Autodesk Inventor part; units mm, degrees
(part 2 of 2)
sketch "Sketch6" plane through (4200, 27800, -3800) normal (0, 0, 1) x (1, 0, 0)
  line L0 (0, -26000) -> (1000, -26000)
  line L1 (1000, -26000) -> (1000, -26050)
  line L2 (1000, -26050) -> (0, -26050)
  line L3 (0, -26050) -> (0, -26000)
  line L4 (1000, -25800) -> (1300, -25800)
  line L5 (1300, -25800) -> (1300, -25850)
  line L6 (1300, -25850) -> (1000, -25850)
  line L7 (1000, -25850) -> (1000, -25800)
  line L8 (1300, -25600) -> (1600, -25600)
  line L9 (1600, -25600) -> (1600, -25650)
  line L10 (1600, -25650) -> (1300, -25650)
  line L11 (1300, -25650) -> (1300, -25600)
  line L12 (1600, -25400) -> (1900, -25400)
  line L13 (1900, -25400) -> (1900, -25450)
  line L14 (1900, -25450) -> (1600, -25450)
  line L15 (1600, -25450) -> (1600, -25400)
  line L16 (1900, -25200) -> (2200, -25200)
  line L17 (2200, -25200) -> (2200, -25250)
  line L18 (2200, -25250) -> (1900, -25250)
  line L19 (1900, -25250) -> (1900, -25200)
  line L20 (2200, -25000) -> (2500, -25000)
  line L21 (2500, -25000) -> (2500, -25050)
  line L22 (2500, -25050) -> (2200, -25050)
  line L23 (2200, -25050) -> (2200, -25000)
  line L24 (2500, -24800) -> (2800, -24800)
  line L25 (2800, -24800) -> (2800, -24850)
  line L26 (2800, -24850) -> (2500, -24850)
  line L27 (2500, -24850) -> (2500, -24800)
  line L28 (2800, -24600) -> (3100, -24600)
  line L29 (3100, -24600) -> (3100, -24650)
  line L30 (3100, -24650) -> (2800, -24650)
  line L31 (2800, -24650) -> (2800, -24600)
  line L32 (3100, -24400) -> (3400, -24400)
  line L33 (3400, -24400) -> (3400, -24450)
  line L34 (3400, -24450) -> (3100, -24450)
  line L35 (3100, -24450) -> (3100, -24400)
  line L36 (0, -22400) -> (1000, -22400)
  line L37 (1000, -22400) -> (1000, -22450)
  line L38 (1000, -22450) -> (0, -22450)
  line L39 (0, -22450) -> (0, -22400)
  line L40 (1000, -22200) -> (1300, -22200)
  line L41 (1300, -22200) -> (1300, -22250)
  line L42 (1300, -22250) -> (1000, -22250)
  line L43 (1000, -22250) -> (1000, -22200)
  line L44 (1300, -22000) -> (1600, -22000)
  line L45 (1600, -22000) -> (1600, -22050)
  line L46 (1600, -22050) -> (1300, -22050)
  line L47 (1300, -22050) -> (1300, -22000)
  line L48 (1600, -21800) -> (1900, -21800)
  line L49 (1900, -21800) -> (1900, -21850)
  line L50 (1900, -21850) -> (1600, -21850)
  line L51 (1600, -21850) -> (1600, -21800)
  line L52 (1900, -21600) -> (2200, -21600)
  line L53 (2200, -21600) -> (2200, -21650)
  line L54 (2200, -21650) -> (1900, -21650)
  line L55 (1900, -21650) -> (1900, -21600)
  line L56 (2200, -21400) -> (2500, -21400)
  line L57 (2500, -21400) -> (2500, -21450)
  line L58 (2500, -21450) -> (2200, -21450)
  line L59 (2200, -21450) -> (2200, -21400)
  line L60 (2500, -21200) -> (2800, -21200)
  line L61 (2800, -21200) -> (2800, -21250)
  line L62 (2800, -21250) -> (2500, -21250)
  line L63 (2500, -21250) -> (2500, -21200)
  line L64 (2800, -21000) -> (3100, -21000)
  line L65 (3100, -21000) -> (3100, -21050)
  line L66 (3100, -21050) -> (2800, -21050)
  line L67 (2800, -21050) -> (2800, -21000)
  line L68 (3100, -20800) -> (3400, -20800)
  line L69 (3400, -20800) -> (3400, -20850)
  line L70 (3400, -20850) -> (3100, -20850)
  line L71 (3100, -20850) -> (3100, -20800)
  line L72 (0, -19400) -> (1100, -19400)
  line L73 (1100, -19400) -> (1100, -19450)
  line L74 (1100, -19450) -> (0, -19450)
  line L75 (0, -19450) -> (0, -19400)
  line L76 (1100, -19250) -> (1100, -19200)
  line L77 (1400, -19250) -> (1100, -19250)
  line L78 (1100, -19200) -> (1400, -19200)
  line L79 (1400, -19200) -> (1400, -19250)
  line L80 (1400, -19050) -> (1400, -19000)
  line L81 (1700, -19050) -> (1400, -19050)
  line L82 (1400, -19000) -> (1700, -19000)
  line L83 (1700, -19000) -> (1700, -19050)
  line L84 (1700, -18794.0956) -> (1700, -18744.0956)
  line L85 (2000, -18794.0956) -> (1700, -18794.0956)
  line L86 (1700, -18744.0956) -> (2000, -18744.0956)
  line L87 (2000, -18744.0956) -> (2000, -18794.0956)
  line L88 (2000, -18594.0956) -> (2000, -18544.0956)
  line L89 (2300, -18594.0956) -> (2000, -18594.0956)
  line L90 (2000, -18544.0956) -> (2300, -18544.0956)
  line L91 (2300, -18544.0956) -> (2300, -18594.0956)
  line L92 (2300, -18394.0956) -> (2300, -18344.0956)
  line L93 (2600, -18394.0956) -> (2300, -18394.0956)
  line L94 (2300, -18344.0956) -> (2600, -18344.0956)
  line L95 (2600, -18344.0956) -> (2600, -18394.0956)
  line L96 (0, -16800) -> (1100, -16800)
  line L97 (1100, -16800) -> (1100, -16850)
  line L98 (1100, -16850) -> (0, -16850)
  line L99 (0, -16850) -> (0, -16800)
  line L100 (1100, -16650) -> (1100, -16600)
  line L101 (1400, -16650) -> (1100, -16650)
  line L102 (1100, -16600) -> (1400, -16600)
  line L103 (1400, -16600) -> (1400, -16650)
  line L104 (1400, -16450) -> (1400, -16400)
  line L105 (1700, -16450) -> (1400, -16450)
  line L106 (1400, -16400) -> (1700, -16400)
  line L107 (1700, -16400) -> (1700, -16450)
  line L108 (1700, -16194.0956) -> (1700, -16144.0956)
  line L109 (2000, -16194.0956) -> (1700, -16194.0956)
  line L110 (1700, -16144.0956) -> (2000, -16144.0956)
  line L111 (2000, -16144.0956) -> (2000, -16194.0956)
  line L112 (2000, -15994.0956) -> (2000, -15944.0956)
  line L113 (2300, -15994.0956) -> (2000, -15994.0956)
  line L114 (2000, -15944.0956) -> (2300, -15944.0956)
  line L115 (2300, -15944.0956) -> (2300, -15994.0956)
  line L116 (2300, -15794.0956) -> (2300, -15744.0956)
  line L117 (2600, -15794.0956) -> (2300, -15794.0956)
  line L118 (2300, -15744.0956) -> (2600, -15744.0956)
  line L119 (2600, -15744.0956) -> (2600, -15794.0956)
  line L120 (0, -14200) -> (1100, -14200)
  line L121 (1100, -14200) -> (1100, -14250)
  line L122 (1100, -14250) -> (0, -14250)
  line L123 (0, -14250) -> (0, -14200)
  line L124 (1100, -14050) -> (1100, -14000)
  line L125 (1400, -14050) -> (1100, -14050)
  line L126 (1100, -14000) -> (1400, -14000)
  line L127 (1400, -14000) -> (1400, -14050)
  line L128 (1400, -13850) -> (1400, -13800)
  line L129 (1700, -13850) -> (1400, -13850)
  line L130 (1400, -13800) -> (1700, -13800)
  line L131 (1700, -13800) -> (1700, -13850)
  line L132 (1700, -13594.0956) -> (1700, -13544.0956)
  line L133 (2000, -13594.0956) -> (1700, -13594.0956)
  line L134 (1700, -13544.0956) -> (2000, -13544.0956)
  line L135 (2000, -13544.0956) -> (2000, -13594.0956)
  line L136 (2000, -13394.0956) -> (2000, -13344.0956)
  line L137 (2300, -13394.0956) -> (2000, -13394.0956)
  line L138 (2000, -13344.0956) -> (2300, -13344.0956)
  line L139 (2300, -13344.0956) -> (2300, -13394.0956)
  line L140 (2300, -13194.0956) -> (2300, -13144.0956)
  line L141 (2600, -13194.0956) -> (2300, -13194.0956)
  line L142 (2300, -13144.0956) -> (2600, -13144.0956)
  line L143 (2600, -13144.0956) -> (2600, -13194.0956)
  line L144 (0, -11600) -> (1100, -11600)
  line L145 (1100, -11600) -> (1100, -11650)
  line L146 (1100, -11650) -> (0, -11650)
  line L147 (0, -11650) -> (0, -11600)
  line L148 (1100, -11450) -> (1100, -11400)
  line L149 (1400, -11450) -> (1100, -11450)
  line L150 (1100, -11400) -> (1400, -11400)
  line L151 (1400, -11400) -> (1400, -11450)
  line L152 (1400, -11250) -> (1400, -11200)
  line L153 (1700, -11250) -> (1400, -11250)
  line L154 (1400, -11200) -> (1700, -11200)
  line L155 (1700, -11200) -> (1700, -11250)
  line L156 (1700, -10994.0956) -> (1700, -10944.0956)
  line L157 (2000, -10994.0956) -> (1700, -10994.0956)
  line L158 (1700, -10944.0956) -> (2000, -10944.0956)
  line L159 (2000, -10944.0956) -> (2000, -10994.0956)
  line L160 (2000, -10794.0956) -> (2000, -10744.0956)
  line L161 (2300, -10794.0956) -> (2000, -10794.0956)
  line L162 (2000, -10744.0956) -> (2300, -10744.0956)
  line L163 (2300, -10744.0956) -> (2300, -10794.0956)
  line L164 (2300, -10594.0956) -> (2300, -10544.0956)
  line L165 (2600, -10594.0956) -> (2300, -10594.0956)
  line L166 (2300, -10544.0956) -> (2600, -10544.0956)
  line L167 (2600, -10544.0956) -> (2600, -10594.0956)
  line L168 (1700, -8650) -> (1400, -8650)
  line L169 (1700, -8600) -> (1700, -8650)
  line L170 (1400, -8650) -> (1400, -8600)
  line L171 (1400, -8600) -> (1700, -8600)
  line L172 (2000, -8394.0956) -> (1700, -8394.0956)
  line L173 (2000, -8344.0956) -> (2000, -8394.0956)
  line L174 (1700, -8394.0956) -> (1700, -8344.0956)
  line L175 (1700, -8344.0956) -> (2000, -8344.0956)
  line L176 (2000, -8194.0956) -> (2000, -8144.0956)
  line L177 (2300, -8194.0956) -> (2000, -8194.0956)
  line L178 (2000, -8144.0956) -> (2300, -8144.0956)
  line L179 (2300, -8144.0956) -> (2300, -8194.0956)
  line L180 (2300, -7994.0956) -> (2300, -7944.0956)
  line L181 (2300, -7944.0956) -> (2600, -7944.0956)
  line L182 (2600, -7944.0956) -> (2600, -7994.0956)
  line L183 (2600, -7994.0956) -> (2300, -7994.0956)
  line L184 (1400, -8800) -> (1400, -8850)
  line L185 (1100, -8800) -> (1400, -8800)
  line L186 (1100, -8850) -> (1100, -8800)
  line L187 (1400, -8850) -> (1100, -8850)
  line L188 (1100, -9000) -> (1100, -9050)
  line L189 (0, -9000) -> (1100, -9000)
  line L190 (1100, -9050) -> (0, -9050)
  line L191 (0, -9050) -> (0, -9000)
  line L192 (1700, -6050) -> (1400, -6050)
  line L193 (1700, -6000) -> (1700, -6050)
  line L194 (1400, -6050) -> (1400, -6000)
  line L195 (1400, -6000) -> (1700, -6000)
  line L196 (2000, -5794.0956) -> (1700, -5794.0956)
  line L197 (2000, -5744.0956) -> (2000, -5794.0956)
  line L198 (1700, -5794.0956) -> (1700, -5744.0956)
  line L199 (1700, -5744.0956) -> (2000, -5744.0956)
  line L200 (2000, -5594.0956) -> (2000, -5544.0956)
  line L201 (2300, -5594.0956) -> (2000, -5594.0956)
  line L202 (2000, -5544.0956) -> (2300, -5544.0956)
  line L203 (2300, -5544.0956) -> (2300, -5594.0956)
  line L204 (2300, -5394.0956) -> (2300, -5344.0956)
  line L205 (2300, -5344.0956) -> (2600, -5344.0956)
  line L206 (2600, -5344.0956) -> (2600, -5394.0956)
  line L207 (2600, -5394.0956) -> (2300, -5394.0956)
  line L208 (1400, -6200) -> (1400, -6250)
  line L209 (1100, -6200) -> (1400, -6200)
  line L210 (1100, -6250) -> (1100, -6200)
  line L211 (1400, -6250) -> (1100, -6250)
  line L212 (1100, -6400) -> (1100, -6450)
  line L213 (0, -6400) -> (1100, -6400)
  line L214 (1100, -6450) -> (0, -6450)
  line L215 (0, -6450) -> (0, -6400)
  line L216 (1700, -3450) -> (1400, -3450)
  line L217 (1700, -3400) -> (1700, -3450)
  line L218 (1400, -3450) -> (1400, -3400)
  line L219 (1400, -3400) -> (1700, -3400)
  line L220 (2000, -3194.0956) -> (1700, -3194.0956)
  line L221 (2000, -3144.0956) -> (2000, -3194.0956)
  line L222 (1700, -3194.0956) -> (1700, -3144.0956)
  line L223 (1700, -3144.0956) -> (2000, -3144.0956)
  line L224 (2000, -2994.0956) -> (2000, -2944.0956)
  line L225 (2300, -2994.0956) -> (2000, -2994.0956)
  line L226 (2000, -2944.0956) -> (2300, -2944.0956)
  line L227 (2300, -2944.0956) -> (2300, -2994.0956)
  line L228 (2300, -2794.0956) -> (2300, -2744.0956)
  line L229 (2300, -2744.0956) -> (2600, -2744.0956)
  line L230 (2600, -2744.0956) -> (2600, -2794.0956)
  line L231 (2600, -2794.0956) -> (2300, -2794.0956)
  line L232 (1400, -3600) -> (1400, -3650)
  line L233 (1100, -3600) -> (1400, -3600)
  line L234 (1100, -3650) -> (1100, -3600)
  line L235 (1400, -3650) -> (1100, -3650)
  line L236 (1100, -3800) -> (1100, -3850)
  line L237 (0, -3800) -> (1100, -3800)
  line L238 (1100, -3850) -> (0, -3850)
  line L239 (0, -3850) -> (0, -3800)
  point P0 (-4200, -27800)
  dimension "d407" = 4200
  dimension "d408" = 1800
  dimension "d409" = 50
  dimension "d410" = 1000
  dimension "d411" = 50
  dimension "d412" = 0
  dimension "d413" = 200
  dimension "d414" = 50
  dimension "d415" = 50
  dimension "d416" = 50
  dimension "d417" = 50
  dimension "d418" = 50
  dimension "d419" = 50
  dimension "d420" = 50
  dimension "d421" = 200
  dimension "d422" = 0
  dimension "d423" = 300
  dimension "d424" = 300
  dimension "d425" = 0
  dimension "d426" = 200
  dimension "d427" = 300
  dimension "d428" = 300
  dimension "d429" = 200
  dimension "d430" = 300
  dimension "d431" = 0
  dimension "d432" = 200
  dimension "d433" = 300
  dimension "d434" = 200
  dimension "d435" = 0
  dimension "d436" = 300
  dimension "d437" = 200
  dimension "d438" = 0
  dimension "d439" = 300
  dimension "d440" = 0
  dimension "d441" = 200
  dimension "d442" = 300
  dimension "d443" = 50
  dimension "d444" = 1000
  dimension "d445" = 50
  dimension "d446" = 0
  dimension "d447" = 200
  dimension "d448" = 50
  dimension "d449" = 50
  dimension "d450" = 50
  dimension "d451" = 50
  dimension "d452" = 50
  dimension "d453" = 50
  dimension "d454" = 50
  dimension "d455" = 200
  dimension "d456" = 0
  dimension "d457" = 300
  dimension "d458" = 300
  dimension "d459" = 0
  dimension "d460" = 200
  dimension "d461" = 300
  dimension "d462" = 300
  dimension "d463" = 200
  dimension "d464" = 300
  dimension "d465" = 0
  dimension "d466" = 200
  dimension "d467" = 300
  dimension "d468" = 200
  dimension "d469" = 0
  dimension "d470" = 300
  constraints: 480 end point, 120 parallel, 60 horizontal, 60 perpendicular
  measures "d407" distance from line of point (-4200, -27800) L3
  measures "d408" distance from line of point (-4200, -27800) L0
  measures "d409" distance between parallel lines of L2 L0
  measures "d410" distance between parallel lines of L3 L1
  measures "d411" distance between parallel lines of L6 L4
  measures "d412" distance between parallel lines of L1 L7
  measures "d413" distance between parallel lines of L0 L4
  measures "d414" distance between parallel lines of L10 L8
  measures "d415" distance between parallel lines of L14 L12
  measures "d416" distance between parallel lines of L18 L16
  measures "d417" distance between parallel lines of L22 L20
  measures "d418" distance between parallel lines of L26 L24
  measures "d419" distance between parallel lines of L30 L28
  measures "d420" distance between parallel lines of L34 L32
  measures "d421" distance between parallel lines of L4 L8
  measures "d422" distance between parallel lines of L5 L11
  measures "d423" distance between parallel lines of L5 L9
  measures "d424" distance between parallel lines of L7 L11
  measures "d425" distance between parallel lines of L9 L15
  measures "d426" distance between parallel lines of L8 L12
  measures "d427" distance between parallel lines of L15 L19
  measures "d428" distance between parallel lines of L9 L13
  measures "d429" distance between parallel lines of L12 L16
  measures "d430" distance between parallel lines of L13 L17
  measures "d431" distance between parallel lines of L17 L23
  measures "d432" distance between parallel lines of L16 L20
  measures "d433" distance between parallel lines of L17 L21
  measures "d434" distance between parallel lines of L20 L24
  measures "d435" distance between parallel lines of L21 L27
  measures "d436" distance between parallel lines of L21 L25
  measures "d437" distance between parallel lines of L24 L28
  measures "d438" distance between parallel lines of L25 L31
  measures "d439" distance between parallel lines of L25 L29
  measures "d440" distance between parallel lines of L35 L29
  measures "d441" distance between parallel lines of L28 L32
  measures "d442" distance between parallel lines of L29 L33
  measures "d443" distance between parallel lines of L38 L36
  measures "d444" distance between parallel lines of L39 L37
  measures "d445" distance between parallel lines of L42 L40
  measures "d446" distance between parallel lines of L37 L43
  measures "d447" distance between parallel lines of L36 L40
  measures "d448" distance between parallel lines of L46 L44
  measures "d449" distance between parallel lines of L50 L48
  measures "d450" distance between parallel lines of L54 L52
  measures "d451" distance between parallel lines of L58 L56
  measures "d452" distance between parallel lines of L62 L60
  measures "d453" distance between parallel lines of L66 L64
  measures "d454" distance between parallel lines of L70 L68
  measures "d455" distance between parallel lines of L40 L44
  measures "d456" distance between parallel lines of L41 L47
  measures "d457" distance between parallel lines of L41 L45
  measures "d458" distance between parallel lines of L43 L47
  measures "d459" distance between parallel lines of L45 L51
  measures "d460" distance between parallel lines of L44 L48
  measures "d461" distance between parallel lines of L51 L55
  measures "d462" distance between parallel lines of L45 L49
  measures "d463" distance between parallel lines of L48 L52
  measures "d464" distance between parallel lines of L49 L53
  measures "d465" distance between parallel lines of L53 L59
  measures "d466" distance between parallel lines of L52 L56
  measures "d467" distance between parallel lines of L53 L57
  measures "d468" distance between parallel lines of L56 L60
  measures "d469" distance between parallel lines of L57 L63
  measures "d470" distance between parallel lines of L57 L61
extrude "Extrusion21" add sketch "Sketch6" along normal blind 1200 and the other way blind 100 contours L0 L1 L2 L3 | L36 L37 L38 L39 | L72 L73 L74 L75 | L96 L97 L98 L99 | L120 L121 L122 L123 | L144 L145 L146 L147 | L188 L190 L191 L189 | L212 L214 L215 L213 | L236 L238 L239 L237
extrude "Extrusion22" add sketch "Sketch6" along normal blind 1200 contours L4 L5 L6 L7 | L8 L9 L10 L11 | L12 L13 L14 L15 | L16 L17 L18 L19 | L20 L21 L22 L23 | L24 L25 L26 L27 | L28 L29 L30 L31 | L32 L33 L34 L35 | L40 L41 L42 L43 | L44 L45 L46 L47 | L48 L49 L50 L51 | L52 L53 L54 L55 | L56 L57 L58 L59 | L60 L61 L62 L63 | L64 L65 L66 L67 | L68 L69 L70 L71 | L76 L78 L79 L77 | L80 L82 L83 L81 | L84 L86 L87 L85 | L88 L90 L91 L89 | L92 L94 L95 L93 | L100 L102 L103 L101 | L104 L106 L107 L105 | L108 L110 L111 L109 | L112 L114 L115 L113 | L116 L118 L119 L117 | L124 L126 L127 L125 | L128 L130 L131 L129 | L132 L134 L135 L133 | L136 L138 L139 L137 | L140 L142 L143 L141 | L148 L150 L151 L149 | L152 L154 L155 L153 | L156 L158 L159 L157 | L160 L162 L163 L161 | L164 L166 L167 L165 | L168 L170 L171 L169 | L172 L174 L175 L173 | L176 L178 L179 L177 | L180 L181 L182 L183 | L184 L187 L186 L185 | L192 L194 L195 L193 | L196 L198 L199 L197 | L200 L202 L203 L201 | L204 L205 L206 L207 | L208 L211 L210 L209 | L216 L218 L219 L217 | L220 L222 L223 L221 | L224 L226 L227 L225 | L228 L229 L230 L231 | L232 L235 L234 L233
sketch "Sketch7" plane through (11900, 0, -2400) normal (1, 0, 0) x (0, 0, -1)
  line L0 (0, 0) -> (6500, 0) projected
  line L1 (200, 2100) -> (1100, 2100)
  line L2 (1100, 2100) -> (1100, 0)
  line L3 (1100, 0) -> (200, 0)
  line L4 (200, 0) -> (200, 2100)
  line L5 (200, 5700) -> (1100, 5700)
  line L6 (1100, 5700) -> (1100, 3600)
  line L7 (1100, 3600) -> (200, 3600)
  line L8 (200, 3600) -> (200, 5700)
  line L9 (200, 9300) -> (1100, 9300)
  line L10 (1100, 9300) -> (1100, 7200)
  line L11 (1100, 7200) -> (200, 7200)
  line L12 (200, 7200) -> (200, 9300)
  line L13 (200, 11900) -> (1100, 11900)
  line L14 (1100, 11900) -> (1100, 9800)
  line L15 (1100, 9800) -> (200, 9800)
  line L16 (200, 9800) -> (200, 11900)
  line L17 (200, 14500) -> (1100, 14500)
  line L18 (1100, 14500) -> (1100, 12400)
  line L19 (1100, 12400) -> (200, 12400)
  line L20 (200, 12400) -> (200, 14500)
  line L21 (200, 17100) -> (1100, 17100)
  line L22 (1100, 17100) -> (1100, 15000)
  line L23 (1100, 15000) -> (200, 15000)
  line L24 (200, 15000) -> (200, 17100)
  line L25 (200, 19700) -> (1100, 19700)
  line L26 (1100, 19700) -> (1100, 17600)
  line L27 (1100, 17600) -> (200, 17600)
  line L28 (200, 17600) -> (200, 19700)
  line L29 (200, 22300) -> (1100, 22300)
  line L30 (1100, 22300) -> (1100, 20200)
  line L31 (1100, 20200) -> (200, 20200)
  line L32 (200, 20200) -> (200, 22300)
  line L33 (200, 24900) -> (1100, 24900)
  line L34 (1100, 24900) -> (1100, 22800)
  line L35 (1100, 22800) -> (200, 22800)
  line L36 (200, 22800) -> (200, 24900)
  line L37 (200, 27500) -> (1100, 27500)
  line L38 (1100, 27500) -> (1100, 25400)
  line L39 (1100, 25400) -> (200, 25400)
  line L40 (200, 25400) -> (200, 27500)
  point P0 (-2400, 0)
  dimension "d653" = 2600
  dimension "d654" = 0
  dimension "d655" = 2100
  dimension "d656" = 900
  dimension "d657" = 900
  dimension "d658" = 1500
  dimension "d659" = 900
  dimension "d660" = 2100
  dimension "d661" = 900
  dimension "d662" = 2100
  dimension "d663" = 900
  dimension "d664" = 2100
  dimension "d665" = 900
  dimension "d666" = 2100
  dimension "d667" = 900
  dimension "d668" = 2100
  dimension "d669" = 900
  dimension "d670" = 2100
  dimension "d671" = 900
  dimension "d672" = 2100
  dimension "d673" = 900
  dimension "d674" = 2100
  dimension "d675" = 900
  dimension "d676" = 2100
  dimension "d677" = 7200
  dimension "d678" = 2600
  dimension "d679" = 2600
  dimension "d680" = 900
  dimension "d681" = 2600
  dimension "d682" = 900
  dimension "d683" = 2600
  dimension "d684" = 900
  dimension "d685" = 2600
  dimension "d686" = 900
  dimension "d687" = 2600
  dimension "d688" = 900
  dimension "d689" = 2600
  dimension "d690" = 900
  dimension "d691" = 2600
  dimension "d692" = 900
  dimension "d693" = 900
  constraints: 80 end point, 20 parallel, 10 horizontal, 10 perpendicular
  measures "d653" distance from line of L4 point (-2400, 0)
  measures "d654" distance from line of point (-2400, 0) L3
  measures "d655" distance between parallel lines of L0 L1
  measures "d656" distance between parallel lines of L2 L4
  measures "d657" distance between parallel lines of L6 L8
  measures "d658" distance between parallel lines of L1 L7
  measures "d659" distance between parallel lines of L4 L6
  measures "d660" distance between parallel lines of L5 L7
  measures "d661" distance between parallel lines of L10 L12
  measures "d662" distance between parallel lines of L9 L11
  measures "d663" distance between parallel lines of L14 L16
  measures "d664" distance between parallel lines of L13 L15
  measures "d665" distance between parallel lines of L18 L20
  measures "d666" distance between parallel lines of L17 L19
  measures "d667" distance between parallel lines of L22 L24
  measures "d668" distance between parallel lines of L21 L23
  measures "d669" distance between parallel lines of L26 L28
  measures "d670" distance between parallel lines of L25 L27
  measures "d671" distance between parallel lines of L30 L32
  measures "d672" distance between parallel lines of L29 L31
  measures "d673" distance between parallel lines of L34 L36
  measures "d674" distance between parallel lines of L33 L35
  measures "d675" distance between parallel lines of L38 L40
  measures "d676" distance between parallel lines of L37 L39
  measures "d677" distance from line of point (-2400, 0) L11
  measures "d678" distance from line of point (-2400, 0) L12
  measures "d679" distance between parallel lines of L9 L13
  measures "d680" distance between parallel lines of L10 L16
  measures "d681" distance between parallel lines of L17 L13
  measures "d682" distance between parallel lines of L14 L20
  measures "d683" distance between parallel lines of L21 L17
  measures "d684" distance between parallel lines of L18 L24
  measures "d685" distance between parallel lines of L21 L25
  measures "d686" distance between parallel lines of L22 L28
  measures "d687" distance between parallel lines of L25 L29
  measures "d688" distance between parallel lines of L26 L32
  measures "d689" distance between parallel lines of L29 L33
  measures "d690" distance between parallel lines of L30 L36
  measures "d691" distance between parallel lines of L33 L37
  measures "d692" distance between parallel lines of L34 L40
  measures "d693" distance between parallel lines of L6 L12
extrude "Extrusion23" cut sketch "Sketch7" against normal blind 200 contours L4 L1 L2 L0
extrude "Extrusion24" cut sketch "Sketch7" against normal blind 200 contours L5 L6 L7 L8
extrude "Extrusion25" cut sketch "Sketch7" against normal blind 200 contours L9 L10 L11 L12 | L13 L14 L15 L16 | L17 L18 L19 L20 | L21 L22 L23 L24 | L25 L26 L27 L28 | L29 L30 L31 L32 | L33 L34 L35 L36 | L37 L38 L39 L40
sketch "Sketch9" plane through (4200, 27800, -3900) normal (0, 0, 1) x (1, 0, 0)
  line L0 (0, -24200) -> (3400, -24200)
  line L1 (3400, -24200) -> (3400, -24400)
  line L2 (3400, -24400) -> (0, -24400)
  line L3 (0, -24400) -> (0, -24200)
  point P0 (-4200, -27800)
  dimension "d742" = 4200
  dimension "d743" = 3400
  dimension "d744" = 200
  dimension "d745" = 3400
  constraints: 8 end point, 2 parallel, 1 horizontal, 1 perpendicular
  measures "d742" distance from line of point (-4200, -27800) L3
  measures "d743" distance from line of point (-4200, -27800) L2
  measures "d744" distance between parallel lines of L2 L0
  measures "d745" distance between parallel lines of L3 L1
extrude "Extrusion27" cut sketch "Sketch9" along normal blind 1300 and the other way blind 1200
sketch "Sketch10" plane through (4200, 27800, -3900) normal (0, 0, 1) x (1, 0, 0)
  line L0 (0, -20600) -> (3400, -20600)
  line L1 (3400, -20600) -> (3400, -20800)
  line L2 (3400, -20800) -> (0, -20800)
  line L3 (0, -20800) -> (0, -20600)
  line L4 (0, -18000) -> (2600, -18000)
  line L5 (2600, -18000) -> (2600, -18200)
  line L6 (2600, -18200) -> (0, -18200)
  line L7 (0, -18200) -> (0, -18000)
  line L8 (0, -15400) -> (2600, -15400)
  line L9 (2600, -15400) -> (2600, -15600)
  line L10 (2600, -15600) -> (0, -15600)
  line L11 (0, -15600) -> (0, -15400)
  line L12 (0, -12800) -> (2600, -12800)
  line L13 (2600, -12800) -> (2600, -13000)
  line L14 (2600, -13000) -> (0, -13000)
  line L15 (0, -13000) -> (0, -12800)
  line L16 (0, -10200) -> (2600, -10200)
  line L17 (2600, -10200) -> (2600, -10400)
  line L18 (2600, -10400) -> (0, -10400)
  line L19 (0, -10400) -> (0, -10200)
  line L20 (0, -7600) -> (2600, -7600)
  line L21 (2600, -7600) -> (2600, -7800)
  line L22 (2600, -7800) -> (0, -7800)
  line L23 (0, -7800) -> (0, -7600)
  line L24 (0, -5000) -> (2600, -5000)
  line L25 (2600, -5000) -> (2600, -5200)
  line L26 (2600, -5200) -> (0, -5200)
  line L27 (0, -5200) -> (0, -5000)
  line L28 (0, -2400) -> (2600, -2400)
  line L29 (2600, -2400) -> (2600, -2600)
  line L30 (2600, -2600) -> (0, -2600)
  line L31 (0, -2600) -> (0, -2400)
  point P0 (-4200, -27800)
  dimension "d750" = 200
  dimension "d751" = 4200
  dimension "d752" = 3400
  dimension "d753" = 7200
  dimension "d754" = 4200
  dimension "d755" = 2600
  dimension "d756" = 2600
  dimension "d757" = 200
  dimension "d758" = 2600
  dimension "d759" = 200
  dimension "d760" = 2600
  dimension "d761" = 200
  dimension "d762" = 2600
  dimension "d763" = 200
  dimension "d764" = 2600
  dimension "d765" = 2600
  dimension "d766" = 2600
  dimension "d767" = 2600
  dimension "d768" = 2600
  dimension "d769" = 2600
  dimension "d770" = 2600
  dimension "d771" = 200
  dimension "d772" = 2600
  dimension "d773" = 200
  dimension "d774" = 2600
  dimension "d775" = 200
  dimension "d776" = 2600
  dimension "d777" = 2600
  dimension "d778" = 2600
  dimension "d779" = 2600
  dimension "d780" = 2600
  dimension "d781" = 2600
  constraints: 64 end point, 16 parallel, 8 horizontal, 8 perpendicular
  measures "d750" distance between parallel lines of L2 L0
  measures "d751" distance from line of point (-4200, -27800) L3
  measures "d752" distance between parallel lines of L3 L1
  measures "d753" distance from line of point (-4200, -27800) L0
  measures "d754" distance from line of L7 point (-4200, -27800)
  measures "d755" distance between parallel lines of L5 L7
  measures "d756" distance between parallel lines of L0 L4
  measures "d757" distance between parallel lines of L6 L4
  measures "d758" distance between parallel lines of L9 L11
  measures "d759" distance between parallel lines of L10 L8
  measures "d760" distance between parallel lines of L13 L15
  measures "d761" distance between parallel lines of L14 L12
  measures "d762" distance between parallel lines of L17 L19
  measures "d763" distance between parallel lines of L18 L16
  measures "d764" distance between parallel lines of L6 L10
  measures "d765" distance between parallel lines of L7 L9
  measures "d766" distance between parallel lines of L10 L14
  measures "d767" distance between parallel lines of L11 L13
  measures "d768" distance between parallel lines of L14 L18
  measures "d769" distance between parallel lines of L15 L17
  measures "d770" distance between parallel lines of L21 L23
  measures "d771" distance between parallel lines of L22 L20
  measures "d772" distance between parallel lines of L25 L27
  measures "d773" distance between parallel lines of L26 L24
  measures "d774" distance between parallel lines of L29 L31
  measures "d775" distance between parallel lines of L30 L28
  measures "d776" distance between parallel lines of L18 L22
  measures "d777" distance between parallel lines of L19 L21
  measures "d778" distance between parallel lines of L22 L26
  measures "d779" distance between parallel lines of L23 L25
  measures "d780" distance between parallel lines of L26 L30
  measures "d781" distance between parallel lines of L27 L29
extrude "Extrusion28" cut sketch "Sketch10" along normal blind 1300 and the other way blind 1200
sketch "Sketch11" plane through (9400, 15000, -2600) normal (1, 0, 0) x (0, 0, -1)
  line L0 (0, -12900) -> (900, -12900)
  line L1 (900, -12900) -> (900, -15000)
  line L2 (900, -15000) -> (0, -15000)
  line L3 (0, -15000) -> (0, -12900)
  line L4 (0, -9300) -> (900, -9300)
  line L5 (900, -9300) -> (900, -11400)
  line L6 (900, -11400) -> (0, -11400)
  line L7 (0, -11400) -> (0, -9300)
  line L8 (0, -3100) -> (900, -3100)
  line L9 (900, -3100) -> (900, -5200)
  line L10 (900, -5200) -> (0, -5200)
  line L11 (0, -5200) -> (0, -3100)
  line L12 (0, 2100) -> (900, 2100)
  line L13 (900, 2100) -> (900, 0)
  line L14 (900, 0) -> (0, 0)
  line L15 (0, 0) -> (0, 2100)
  line L16 (0, 7300) -> (900, 7300)
  line L17 (900, 7300) -> (900, 5200)
  line L18 (900, 5200) -> (0, 5200)
  line L19 (0, 5200) -> (0, 7300)
  line L20 (0, 12500) -> (900, 12500)
  line L21 (900, 12500) -> (900, 10400)
  line L22 (900, 10400) -> (0, 10400)
  line L23 (0, 10400) -> (0, 12500)
  point P0 (-2600, -15000)
  dimension "d786" = 2100
  dimension "d787" = 2100
  dimension "d788" = 2600
  dimension "d789" = 900
  dimension "d790" = 2100
  dimension "d791" = 900
  dimension "d792" = 2100
  dimension "d793" = 900
  dimension "d794" = 1500
  dimension "d795" = 900
  dimension "d796" = 6200
  dimension "d797" = 900
  dimension "d798" = 2100
  dimension "d799" = 900
  dimension "d800" = 2100
  dimension "d801" = 900
  dimension "d802" = 2100
  dimension "d803" = 900
  dimension "d804" = 5200
  dimension "d805" = 900
  dimension "d806" = 5200
  dimension "d807" = 900
  dimension "d808" = 5200
  dimension "d809" = 900
  constraints: 48 end point, 12 parallel, 6 horizontal, 6 perpendicular
  measures "d786" distance from line of point (-2600, -15000) L0
  measures "d787" distance between parallel lines of L2 L0
  measures "d788" distance from line of point (-2600, -15000) L3
  measures "d789" distance between parallel lines of L1 L3
  measures "d790" distance between parallel lines of L6 L4
  measures "d791" distance between parallel lines of L5 L7
  measures "d792" distance between parallel lines of L10 L8
  measures "d793" distance between parallel lines of L9 L11
  measures "d794" distance between parallel lines of L0 L6
  measures "d795" distance between parallel lines of L3 L5
  measures "d796" distance between parallel lines of L10 L6
  measures "d797" distance between parallel lines of L7 L9
  measures "d798" distance between parallel lines of L14 L12
  measures "d799" distance between parallel lines of L13 L15
  measures "d800" distance between parallel lines of L18 L16
  measures "d801" distance between parallel lines of L17 L19
  measures "d802" distance between parallel lines of L22 L20
  measures "d803" distance between parallel lines of L21 L23
  measures "d804" distance between parallel lines of L8 L12
  measures "d805" distance between parallel lines of L11 L13
  measures "d806" distance between parallel lines of L16 L12
  measures "d807" distance between parallel lines of L13 L19
  measures "d808" distance between parallel lines of L20 L16
  measures "d809" distance between parallel lines of L17 L23
extrude "Extrusion29" cut sketch "Sketch11" against normal blind 200
sketch "Sketch12" plane through (15900, 0, -1000) normal (1, 0, 0) x (0, 0, -1)
  line L0 (3400, 2100) -> (5200, 2100)
  line L1 (5200, 2100) -> (5200, 0)
  line L2 (5200, 0) -> (3400, 0)
  line L3 (3400, 0) -> (3400, 2100)
  point P0 (-1000, 0)
  dimension "d812" = 2100
  dimension "d813" = 4400
  dimension "d814" = 1800
  dimension "d815" = 2100
  constraints: 8 end point, 2 parallel, 1 horizontal, 1 perpendicular
  measures "d812" distance from line of point (-1000, 0) L0
  measures "d813" distance from line of point (-1000, 0) L3
  measures "d814" distance between parallel lines of L1 L3
  measures "d815" distance between parallel lines of L2 L0
extrude "Extrusion30" cut sketch "Sketch12" against normal blind 200
sketch "Sketch13" plane through (1000, 0, -1000) normal (0, 0, 1) x (1, 0, 0)
  line L0 (6400, 2100) -> (7300, 2100)
  line L1 (7300, 2100) -> (7300, 0)
  line L2 (7300, 0) -> (6400, 0)
  line L3 (6400, 0) -> (6400, 2100)
  point P0 (-1000, 0)
  dimension "d818" = 7400
  dimension "d819" = 2100
  dimension "d820" = 900
  dimension "d821" = 2100
  constraints: 8 end point, 2 parallel, 1 horizontal, 1 perpendicular
  measures "d818" distance from line of point (-1000, 0) L3
  measures "d819" distance from line of point (-1000, 0) L0
  measures "d820" distance between parallel lines of L1 L3
  measures "d821" distance between parallel lines of L2 L0
extrude "Extrusion31" cut sketch "Sketch13" against normal blind 200
ref_plane "Work Plane3" through (0, 27800, 0) normal (0, 1, 0) x (1, 0, 0)
sketch "Sketch14" plane through (0, 27800, 0) normal (0, 1, 0) x (1, 0, 0)
  line L0 (1000, 1000) -> (15900, 1000)
  line L1 (15900, 1000) -> (15900, 10300)
  line L2 (15900, 10300) -> (1000, 10300)
  line L3 (1000, 10300) -> (1000, 1000)
  point P0 (0, 0)
  dimension "d825" = 1000
  dimension "d826" = 1000
  dimension "d827" = 14900
  dimension "d828" = 9300
  constraints: 8 end point, 2 parallel, 1 horizontal, 1 perpendicular
  measures "d825" distance from line of point (0, 0) L3
  measures "d826" distance from line of point (0, 0) L0
  measures "d827" distance between parallel lines of L1 L3
  measures "d828" distance between parallel lines of L2 L0
extrude "Extrusion32" add sketch "Sketch14" along normal blind 200
ref_plane "Work Plane4" through (0, 0, 0) normal (0, -1, 0) x (1, 0, 0)
sketch "Sketch15" plane through (0, 0, 0) normal (0, -1, 0) x (1, 0, 0)
  line L0 (0, 0) -> (16900, 0)
  line L1 (16900, 0) -> (16900, -11300)
  line L2 (16900, -11300) -> (0, -11300)
  line L3 (0, -11300) -> (0, 0)
  point P0 (0, 0)
  dimension "d832" = 0
  dimension "d833" = 0
  dimension "d834" = 16900
  dimension "d835" = 11300
  constraints: 8 end point, 2 parallel, 1 horizontal, 1 perpendicular
  measures "d832" distance from line of L0 point (0, 0)
  measures "d833" distance from line of point (0, 0) L3
  measures "d834" distance between parallel lines of L1 L3
  measures "d835" distance between parallel lines of L2 L0
extrude "Extrusion33" add sketch "Sketch15" along normal blind 100
body "Solid1"
